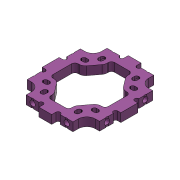
# Autodesk Inventor part: 16_009_COXA_FRAME_4_R1
Saved by Autodesk Inventor 2021.2 (Build 252289000, 289)
## iProperties
Created: 2018-04-27
Part Number: 16_009_COXA_FRAME_4_R1
Material: 一般
Document SubType Name: Modeling
Designer: cmflab
Density: 1 g/cm^3
Appearance: 滑らか - 紫
Mass: 2.23731 g
Surface Area: 27.07 cm^2
Volume: 2.23731 cm^3
Author: cmflab
Autodesk Inventor part; units mm, degrees
ref_plane "YZ Plane" through (0, 0, 0) normal (1, 0, 0) x (0, 1, 0)
ref_plane "XZ Plane" through (0, 0, 0) normal (0, 1, 0) x (-1, 0, 0)
ref_plane "XY Plane" through (0, 0, 0) normal (0, 0, 1) x (1, 0, 0)
sketch "スケッチ1" plane through (0, 0, 0) normal (0, 0, 1) x (1, 0, 0)
  line L0 (0, 0) -> (0, 12.1538) construction
  line L1 (0, 0) -> (23.2096, 0) construction
  arc A0 (7.4, 19) -> (8.6, 19) centre (8, 19.8) ccw
  line L2 (7.4, 19) -> (8.6, 19) construction
  line L3 (8.6, 19) -> (11, 19)
  line L4 (-8, 19.8) -> (8, 19.8) construction
  arc A1 (8.6, -19) -> (7.4, -19) centre (8, -19.8) ccw
  line L5 (7.4, -19) -> (8.6, -19) construction
  line L6 (8.6, -19) -> (11, -19)
  line L7 (-8, -19.8) -> (8, -19.8) construction
  line L8 (17, 12.5) -> (17, 9.6)
  arc A2 (17, 9.6) -> (17, 8.4) centre (17.8, 9) ccw
  arc A3 (17, -8.4) -> (17, -9.6) centre (17.8, -9) ccw
  line L9 (17.8, 9) -> (17.8, -9) construction
  line L10 (17, 8.4) -> (17, 6)
  line L11 (17, 9.6) -> (17, 8.4) construction
  line L12 (17, -8.4) -> (17, -9.6) construction
  line L13 (17, -9.6) -> (17, -12.5)
  line L14 (0, 21) -> (0, 15)
  line L15 (0, -21) -> (3, -21)
  line L16 (3, -21) -> (3, -19)
  line L17 (0, 21) -> (3, 21)
  line L18 (3, 21) -> (3, 19)
  arc A4 (3, 19) -> (5, 19) centre (4, 19) ccw
  arc A5 (5, -19) -> (3, -19) centre (4, -19) ccw
  line L19 (5, -19) -> (7.4, -19)
  line L20 (5, 19) -> (7.4, 19)
  line L21 (11, 19) -> (11, 16.5)
  line L22 (17, 12.5) -> (15, 12.5)
  line L23 (17, -12.5) -> (15, -12.5)
  line L24 (11, -16.5) -> (11, -19)
  arc A6 (11, 16.5) -> (15, 12.5) centre (15, 16.5) ccw
  arc A7 (15, -12.5) -> (11, -16.5) centre (15, -16.5) ccw
  line L25 (7.9, 15) -> (8.1, 15)
  line L26 (9.1, 14) -> (9.1, 13)
  line L27 (8.1, 12) -> (7.9, 12)
  line L28 (6.9, 13) -> (6.9, 14)
  line L29 (11, 10.1) -> (12, 10.1)
  line L30 (13, 9.1) -> (13, 8.9)
  line L31 (12, 7.9) -> (11, 7.9)
  line L32 (10, 8.9) -> (10, 9.1)
  arc A8 (7.9, 15) -> (6.9, 14) centre (7.9, 14) ccw
  arc A9 (9.1, 14) -> (8.1, 15) centre (8.1, 14) ccw
  arc A10 (8.1, 12) -> (9.1, 13) centre (8.1, 13) ccw
  arc A11 (6.9, 13) -> (7.9, 12) centre (7.9, 13) ccw
  arc A12 (11, 10.1) -> (10, 9.1) centre (11, 9.1) ccw
  arc A13 (10, 8.9) -> (11, 7.9) centre (11, 8.9) ccw
  arc A14 (12, 7.9) -> (13, 8.9) centre (12, 8.9) ccw
  arc A15 (13, 9.1) -> (12, 10.1) centre (12, 9.1) ccw
  line L33 (8, 19.8) -> (8, 15) construction
  line L34 (17.8, 9) -> (13, 9) construction
  line L35 (17, 4) -> (18.5, 4)
  line L36 (18.5, 4) -> (18.5, -4)
  line L37 (18.5, -4) -> (17, -4)
  line L38 (17, 4) -> (17, -4) construction
  line L39 (17, -6) -> (17, -8.4)
  arc A16 (17, 6) -> (17, 4) centre (17, 5) ccw
  arc A17 (17, -4) -> (17, -6) centre (17, -5) ccw
  line L40 (0, 15) -> (3.4, 15)
  line L41 (4.9, 13.5) -> (4.9, 13)
  line L42 (5.507, 11.1907) -> (8.607, 7.0907)
  line L43 (11, 5.9) -> (11.5, 5.9)
  line L44 (13, 4.4) -> (13, -4.4)
  arc A18 (4.9, 13) -> (5.507, 11.1907) centre (7.9, 13) ccw
  arc A19 (8.607, 7.0907) -> (11, 5.9) centre (11, 8.9) ccw
  arc A20 (4.9, 13.5) -> (3.4, 15) centre (3.4, 13.5) ccw
  arc A21 (13, 4.4) -> (11.5, 5.9) centre (11.5, 4.4) ccw
  line L45 (0, -15) -> (3.4, -15)
  line L46 (4.9, -13.5) -> (4.9, -13)
  line L47 (5.507, -11.1907) -> (8.607, -7.0907)
  line L48 (11, -5.9) -> (11.5, -5.9)
  arc A22 (5.507, -11.1907) -> (4.9, -13) centre (7.9, -13) ccw
  arc A23 (11, -5.9) -> (8.607, -7.0907) centre (11, -8.9) ccw
  arc A24 (3.4, -15) -> (4.9, -13.5) centre (3.4, -13.5) ccw
  arc A25 (11.5, -5.9) -> (13, -4.4) centre (11.5, -4.4) ccw
  line L49 (0, -15) -> (0, -21)
  line L50 (7.9, -15) -> (8.1, -15)
  line L51 (9.1, -14) -> (9.1, -13)
  line L52 (8.1, -12) -> (7.9, -12)
  line L53 (6.9, -13) -> (6.9, -14)
  line L54 (11, -10.1) -> (12, -10.1)
  line L55 (13, -9.1) -> (13, -8.9)
  line L56 (12, -7.9) -> (11, -7.9)
  line L57 (10, -8.9) -> (10, -9.1)
  arc A26 (6.9, -14) -> (7.9, -15) centre (7.9, -14) ccw
  arc A27 (8.1, -15) -> (9.1, -14) centre (8.1, -14) ccw
  arc A28 (9.1, -13) -> (8.1, -12) centre (8.1, -13) ccw
  arc A29 (7.9, -12) -> (6.9, -13) centre (7.9, -13) ccw
  arc A30 (10, -9.1) -> (11, -10.1) centre (11, -9.1) ccw
  arc A31 (11, -7.9) -> (10, -8.9) centre (11, -8.9) ccw
  arc A32 (13, -8.9) -> (12, -7.9) centre (12, -8.9) ccw
  arc A33 (12, -10.1) -> (13, -9.1) centre (12, -9.1) ccw
  point P0 (0, -12.1538)
  point P1 (8, -15)
  point P2 (13, -9)
  dimension "d4" = 16
  dimension "d6" = 25
  dimension "d7" = 34
  dimension "d8" = 0.8
  dimension "d10" = 1
  dimension "d11" = 18
  dimension "d27" = 6
  dimension "d28" = 1
  dimension "d29" = 2
  dimension "d30" = 38
  dimension "d31" = 22
  dimension "d32" = 0.8
  dimension "d33" = 1
  dimension "d34" = 6
  dimension "d35" = 2
  dimension "d36" = 1
  dimension "d37" = 4
  dimension "d38" = 1
  dimension "d39" = 4
  dimension "d40" = 3
  dimension "d41" = 2.2
  dimension "d42" = 2.2
  dimension "d43" = 4
  dimension "d44" = 3
  dimension "d45" = 1.5
  dimension "d46" = 8
  dimension "d47" = 1
  dimension "d48" = 3
  dimension "d49" = 1.5
  constraints: 116 end point, 68 point on circle, 49 symmetric about line, 34 centre point, 31 tangent, 13 horizontal, 12 equal radius, 10 perpendicular, 7 collinear, 6 parallel, 6 point on line, 6 vertical, 2 concentric, 2 midpoint, 15 other
  measures "d4" distance of L4.start L4.end
  measures "d6" distance of L8.start L13.end
  measures "d7" diameter of L8 L0
  measures "d8" distance between parallel lines of L9 L8
  measures "d10" radius of A2
  measures "d11" distance of L9.start L9.end
  measures "d27" diameter of L18 L0
  measures "d28" radius of A4
  measures "d29" distance between parallel lines of L20 L17
  measures "d30" diameter of L2 L1
  measures "d31" diameter of L3.end L0
  measures "d32" distance between parallel lines of L4 L2
  measures "d33" radius of A0
  measures "d34" diameter of L16 L0
  measures "d35" distance between parallel lines of L15 L5
  measures "d36" radius of A5
  measures "d37" radius of A6
  measures "d38" radius of A8
  measures "d39" distance between parallel lines of L25 L20
  measures "d40" distance between parallel lines of L27 L25
  measures "d41" distance between parallel lines of L26 L28
  measures "d42" distance between parallel lines of L29 L31
  measures "d43" distance between parallel lines of L8 L30
  measures "d44" distance between parallel lines of L30 L32
  measures "d45" distance between parallel lines of L38 L36
  measures "d46" distance between parallel lines of L37 L35
  measures "d47" radius of A16
  measures "d48" radius of A18
  measures "d49" radius of A20
extrude "押し出し2" add sketch "スケッチ1" along normal blind 4
mirror "ミラー3" about plane through (0, 21, 0) normal (-1, 0, 0) of "押し出し2"
sketch "スケッチ2" plane through (-7.4, 19, 0) normal (0, 1, 0) x (1, 0, 0)
  line L0 (14.8, 0) -> (14.8, -4) construction
  line L1 (16, 0) -> (16, -4) construction
  line L2 (14.8, 0) -> (16, -4) construction
  circle A0 centre (-0.6, -2) radius 1.25
  circle A1 centre (15.4, -2) radius 1.25
  line L3 (-1.2, -4) -> (0, -4) construction
  line L4 (-1.2, 0) -> (-1.2, -4) construction
  line L5 (0, -4) -> (-1.2, 0) construction
  dimension "d20" = 2.5
  constraints: 4 end point, 2 centre point, 2 midpoint, 1 equal radius
  measures "d20" diameter of A0
extrude "押し出し3" cut sketch "スケッチ2" against normal blind 5
mirror "ミラー1" about plane through (0, 0, 0) normal (0, 1, 0) of "押し出し3"
sketch "スケッチ3" plane through (17, -8.4, 0) normal (1, 0, 0) x (0, 0, -1)
  circle A0 centre (-2, 17.4) radius 1.25
  circle A1 centre (-2, -0.6) radius 1.25
  line L0 (0, 16.8) -> (0, 18) construction
  line L1 (0, 18) -> (-4, 16.8) construction
  line L2 (0, -1.2) -> (0, 0) construction
  line L3 (0, -1.2) -> (-4, -1.2) construction
  line L4 (0, 0) -> (-4, -1.2) construction
  point P0 (0, 8.4)
  point P1 (-4, 18)
  point P2 (-4, 0)
  dimension "d23" = 2.5
  constraints: 4 end point, 2 centre point, 2 midpoint, 1 coincident, 1 equal radius
  measures "d23" diameter of A0
extrude "押し出し4" cut sketch "スケッチ3" against normal blind 4
mirror "ミラー2" about plane through (0, 0, 0) normal (1, 0, 0) of "押し出し4"
